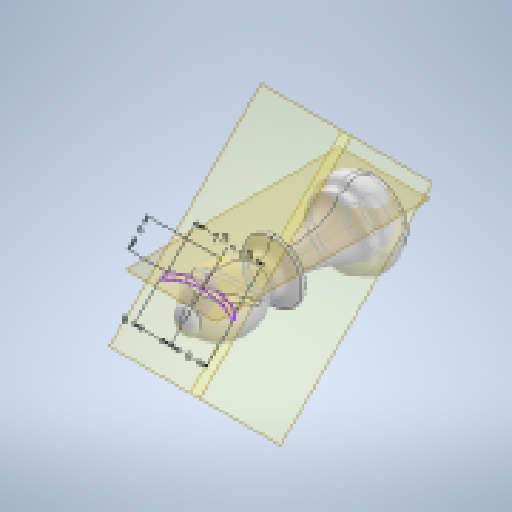
# Autodesk Inventor part: bishop-white
Saved by Autodesk Inventor 2024.1 (Build 281209000, 209)
## iProperties
Created: 2025-08-03
Part Number: bishop-white
Material: Generic
Document SubType Name: Modeling
Designer: iwheard
Density: 1 g/cm^3
Appearance: Default
Author: iwheard
Autodesk Inventor part; units mm, degrees
ref_plane "YZ Plane" through (0, 0, 0) normal (1, 0, 0) x (0, 1, 0)
ref_plane "XY Plane" through (0, 0, 0) normal (0, 0, 1) x (1, 0, 0)
sketch "Sketch1" plane through (0, 0, 0) normal (0, 0, 1) x (1, 0, 0)
  circle A0 centre (0, 25.5) radius 3
  circle A1 centre (0, 25.5) radius 5
  point P0 (0, 0)
  dimension "d0" = 10
  constraints: 2 centre point
  measures "d0" diameter of A1
extrude "Extrusion1" add sketch "Sketch1" along normal blind 3
sketch "Sketch3" plane through (0, 25.5, 3) normal (0, 0, 1) x (1, 0, 0)
  circle A0 centre (0, 0) radius 5 projected
  circle A1 centre (0, 0) radius 3 projected
  circle A2 centre (0, 0) radius 7.15
  point P0 (0, -25.5)
  dimension "d6" = 14.3
  constraints: 1 centre point
  measures "d6" diameter of A2
extrude "Extrusion2" add sketch "Sketch3" against normal blind 3 contours A2
sketch "Sketch2" plane through (0, 0, 0) normal (1, 0, 0) x (0, 1, 0)
  line L0 (30.5, 3) -> (20.5, 3) projected
  line L1 (30.5, 0) -> (20.5, 0) projected
  line L2 (30.5, 0) -> (30.5, 3) projected
  line L3 (28.5, 3) -> (28.5, 0) projected
  line L4 (32.65, 3) -> (18.35, 3) projected
  line L5 (32.65, 3) -> (32.65, 0) projected
  line L6 (28.3472, 21.8) -> (18.9472, 21.8)
  line L7 (19.95, 21.8) -> (32.25, 21.8)
  line L8 (32.65, 0.8) -> (33.5166, 1.2027) construction
  line L9 (33.5166, 1.2027) -> (34.0787, 2.2554) construction
  line L10 (34.0787, 2.2554) -> (34.4911, 4.0365) construction
  line L11 (34.4911, 4.0365) -> (34.2278, 5.2149) construction
  line L12 (34.2278, 5.2149) -> (33.7977, 5.9148) construction
  line L13 (33.7977, 5.9148) -> (33.0833, 6.0655) construction
  line L14 (33.0833, 6.0655) -> (32.65, 6.8872) construction
  line L15 (32.65, 6.8872) -> (33.4405, 8.43) construction
  line L16 (33.4405, 8.43) -> (29.4068, 8.43) construction
  line L17 (29.4068, 8.43) -> (27.9564, 17.9326) construction
  line L18 (32.25, 21.8) -> (32.25, 21.8) construction
  spline S0 degree 4 poles (32.65, 0.8) (33.5166, 1.2027) (34.0787, 2.2554) (34.4911, 4.0365) (34.2278, 5.2149) (33.7977, 5.9148) (33.0833, 6.0655) (32.65, 6.8872) (33.4405, 8.43) (29.4068, 8.43) (27.9564, 17.9326) (28.5, 20.0574) (31.3751, 21.1669) (32.1291, 21.5879) (32.2499, 21.7998) (32.25, 21.8) knots 1 1 1 1 1 2 3 4 5 6 7 8 9 10 10.505813 10.92418 11 11 11 11 11
  ellipse E0 centre (25.5, 41) end of major axis (22.7, 41) minor radius 1.4
  ellipse E1 centre (25.5, 33) end of major axis (25.5, 25) minor radius 6.5
  line L19 (32.25, 21.8) -> (32.4585, 22.7) construction
  line L20 (28.3607, 25.5724) -> (28.3108, 25.7867) construction
  spline S1 degree 4 poles (32.25, 21.8) (32.4585, 22.7) (29.8146, 23.2462) (29.2082, 23.4583) (29.4068, 25.3272) (28.3607, 25.5724) (28.3108, 25.7867) knots 1 1 1 1 1 1.620558 1.874487 2 2 2 2 2
  line L21 (29.4068, 25.3272) -> (28.3607, 25.5724) construction
  line L22 (32.4585, 22.7) -> (29.8146, 23.2462) construction
  line L23 (29.8146, 23.2462) -> (29.2082, 23.4583) construction
  line L24 (29.2082, 23.4583) -> (29.4068, 25.3272) construction
  line L25 (25.5, 42.4) -> (25.5, 3)
  line L26 (32.1291, 21.5879) -> (32.25, 21.8) construction
  line L27 (27.9564, 17.9326) -> (28.5, 20.0574) construction
  line L28 (28.5, 20.0574) -> (31.3751, 21.1669) construction
  line L29 (31.3751, 21.1669) -> (32.1291, 21.5879) construction
  point P0 (0, 0)
  point P1 (25.5, 0)
  point P2 (25.5, 3)
  point P3 (28.01, 40.3795)
  dimension "d127" = 2.8
  dimension "d128" = 1.4
  dimension "d129" = 6.5
  dimension "d130" = 8
  dimension "d89" = 12.3
  dimension "d131" = 8
  dimension "d132" = 33
  dimension "d133" = 11.2
  dimension "d134" = 6.75
  dimension "d135" = 0.8
  constraints: 6 end point, 3 midpoint, 3 vertical alignment, 2 coincident, 1 horizontal, 1 horizontal alignment, 1 point on line, 14 other
  measures "d89" distance of L7.end L7.start
  measures "d131" distance of point (25.5, 33) point (25.5, 41)
  measures "d132" distance from line of L1 point (25.5, 33)
  measures "d133" distance from line of point (25.5, 33) L6
  measures "d134" horizontal distance of point (32.25, 21.8) point (25.5, 33)
  measures "d135" distance from line of L8.start L1
revolve "Revolution1" add sketch "Sketch2" angle 360 about axis through (0, 25.5, 42.4) along (0, 0, -1) picked at (27.4668, 31.4146) picked at (26.1235, 40.0751) picked at (25.9921, 41.4318) contours L0 L25 L6 L7 S0 L5 L4 | L25 E1 S1 L7 L6 | L25 E0 E1 | L25 E1 E0 | E1 L25 E0
fillet "Fillet5" radius 0.6 1 edges at (0, 18.75, 21.8)
ref_plane "Work Plane6" through (0, 32, 33) normal (0, 1, 0) x (-1, 0, 0)
ref_plane "Work Plane9" through (0, 49.6777, 17.6777) normal (0, 0.7071068, 0.7071068) x (1, 0, 0)
ref_plane "Work Plane7" through (0, 32, 0) normal (0, 0.7071068, 0.7071068) x (1, 0, 0)
sketch "Sketch16" plane through (0, 49.6777, 17.6777) normal (0, 0.7071068, 0.7071068) x (1, 0, 0)
  line L0 (8, -30.0355) -> (0, -26.3614) construction
  line L1 (0, -26.3614) -> (-8, -30.0129) construction
  spline S0 degree 2 poles (8, -30.0355) (0, -26.3614) (-8, -30.0129) knots 1 1 1 2 2 2
  line L2 (8, -30.0355) -> (7.5, -28.6475)
  line L3 (-7.5, -28.6274) -> (-8, -30.0129)
  spline S1 degree 5 poles (7.5, -28.6475) (6.0737, -28.0663) (4.5989, -27.6042) (3.0818, -27.2819) (0.0019, -26.958) (-3.0789, -27.2731) (-4.5967, -27.5912) (-6.0725, -28.0496) (-7.5, -28.6274) knots 0 0 0 0 0 0 0.500029 0.500029 0.500029 1 1 1 1 1 1
  point P0 (0, -22.6274)
  point P1 (7.6736, -28.7905)
  point P2 (-7.681, -28.8125)
  point P3 (-4, -29.7611)
  point P4 (4, -29.7611)
  dimension "d137" = 8
  dimension "d138" = 8
  dimension "d141" = 6
  dimension "d142" = 7.5
  dimension "d143" = 7.5
  constraints: 4 end point, 1 vertical alignment, 6 other
  measures "d137" horizontal distance of L1.end point (0, -22.627)
  measures "d138" horizontal distance of L0.start point (0, -22.627)
  measures "d141" vertical distance of point (0, -22.627) L3.start
  measures "d142" horizontal distance of point (0, -22.627) L2.end
  measures "d143" horizontal distance of point (0, -22.627) L3.start
sketch "Sketch17" plane through (0, 0, 0) normal (1, 0, 0) x (0, 1, 0)
  line L0 (29.024, 39.7222) -> (29.1615, 34.9225) construction
  line L1 (29.1615, 34.9225) -> (26.7953, 31.6689) construction
  spline S0 degree 2 poles (29.024, 39.7222) (29.1615, 34.9225) (26.7953, 31.6689) knots 1 1 1 2 2 2
  point P0 (0, 0)
  constraints: 3 other
sweep "Sweep1" cut profiles "Sketch16" path "Sketch17"
body "Solid1"
